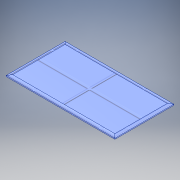
# Autodesk Inventor part: SolarPanel
Saved by Autodesk Inventor 2019 (Build 230136000, 136)
## iProperties
Created: 2018-09-02
Part Number: SolarPanel
Material: Generic
Document SubType Name: Modeling
Designer: Crater-Windows
Density: 1 g/cm^3
Appearance: 4in Square - Light Blue
Author: Crater-Windows
Autodesk Inventor part; units mm, degrees
ref_plane "YZ Plane" through (0, 0, 0) normal (1, 0, 0) x (0, 1, 0)
ref_plane "XZ Plane" through (0, 0, 0) normal (0, 1, 0) x (-1, 0, 0)
ref_plane "XY Plane" through (0, 0, 0) normal (0, 0, 1) x (1, 0, 0)
sketch "Sketch1" plane through (0, 0, 0) normal (0, 1, 0) x (-1, 0, 0)
  line L0 (0, 0) -> (-166, 0)
  line L1 (-166, 0) -> (-166, -90)
  line L2 (-166, -90) -> (0, -90)
  line L3 (0, -90) -> (0, 0)
  dimension "d0" = 166
  dimension "d1" = 90
  constraints: 8 end point, 2 parallel, 1 horizontal, 1 perpendicular
  measures "d0" distance of L2.end L1.end
  measures "d1" distance of L1.end L0.end
extrude "Extrusion1" add sketch "Sketch1" along normal blind 2.54
chamfer "Chamfer1" distance 5 distance2 1 1 edges at (83, 2.54, -90) measured on face at (110.6667, 2.54, -30)
chamfer "Chamfer2" distance 5 distance2 1 1 edges at (0, 2.54, -42.5) measured on face at (110.6667, 2.54, -28.3333)
chamfer "Chamfer3" distance 5 distance2 1 1 edges at (85.5, 2.54, 0) measured on face at (58.6667, 2.54, -56.6667)
chamfer "Chamfer4" distance 5 distance2 1 1 edges at (166, 2.54, -45) measured on face at (112.3333, 2.54, -31.6667)
body "Solid1"
